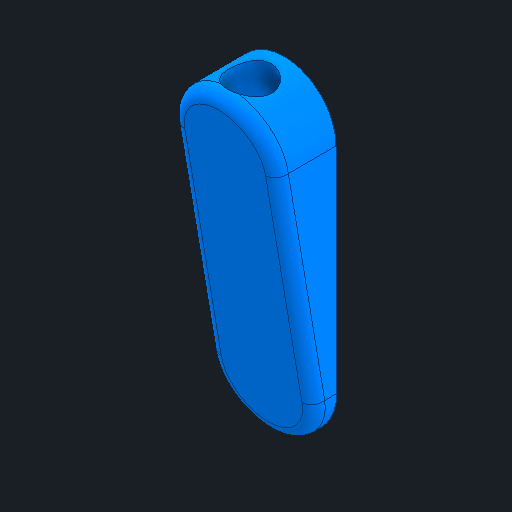
# Autodesk Inventor part: shaft_outlet
Saved by Autodesk Inventor 2023 (Build 270158030, 158C)
## iProperties
Created: 2022-03-28
Part Number: shaft_outlet
Material: Generic
Document SubType Name: Modeling
Designer: kardo
Density: 1 g/cm^3
Appearance: Blue Plastic
Author: kardo
Autodesk Inventor part; units mm, degrees
ref_plane "YZ Plane" through (0, 0, 0) normal (1, 0, 0) x (0, 1, 0)
ref_plane "XZ Plane" through (0, 0, 0) normal (0, 1, 0) x (-1, 0, 0)
ref_plane "XY Plane" through (0, 0, 0) normal (0, 0, 1) x (1, 0, 0)
derived "stencil_frame.ipt"
sketch "sk_drivetrain_profile" plane through (6, 0, 0) normal (1, 0, 0) x (0, 1, 0)
  line L0 (-547.3485, 0) -> (393.091, 0) construction
  line L1 (-363, 4666.1952) -> (-363, -2045.0469) construction
  line L2 (0, 4666.1952) -> (0, -2045.0469) construction
  line L3 (-140.6277, 54.4571) -> (-133.8539, 27.2888)
  line L4 (-395, 0) -> (-331.1194, 3.9071)
  line L5 (-137.2408, 40.8729) -> (-228.5101, 18.117)
  line L6 (-314.0499, 4.9511) -> (-270.6751, 7.604) construction
  line L7 (-270.6751, 7.604) -> (-228.5101, 18.117) construction
  line L8 (-133.8539, 27.2888) -> (-133.8539, 22.2888) construction
  line L9 (-331.1194, 3.9071) -> (-314.0499, 4.9511)
  line L10 (-1246.9714, 4491.7596) -> (383.4376, -2047.4538) construction
  spline S0 degree 2 poles (-314.0499, 4.9511) (-270.6751, 7.604) (-228.5101, 18.117) knots 1 1 1 2 2 2
  line L11 (-229.1821, 20.8126) -> (-137.9129, 43.5685) construction
  line L12 (-136.5687, 38.1773) -> (-227.838, 15.4214) construction
  line L13 (-229.1821, 20.8126) -> (-227.838, 15.4214) construction
  line L14 (0, 21.4767) -> (-254.1001, 20.7404) construction
  line L15 (-55.6943, 22.5153) -> (-309.842, 21.7788) construction
  point P0 (0, 0)
  point P1 (-217.5636, 20.8462)
  point P2 (-205.945, 20.8799)
  point P3 (-201.0754, 22.094)
sketch "sk_prop_shaft_cut" plane through (6, 0, 21.4767) normal (0, -0.0028978, 0.9999958) x (0, -0.9999958, -0.0028978)
  line L0 (229.1831, -4.7781) -> (201.0728, -4.7781)
  line L1 (229.1831, 4.7781) -> (201.0728, 4.7781)
  arc A0 (201.0728, 4.7781) -> (201.0728, -4.7781) centre (201.0728, 0) ccw
  arc A1 (229.1831, -4.7781) -> (229.1831, 4.7781) centre (229.1831, 0) ccw
  point P0 (0.0622, -6)
  point P1 (217.5645, 0)
  point P2 (205.9458, 0)
ref_plane "plane_motor_mount" through (0, -127.05, 0) normal (0, 0.9702957, 0.2419219) x (-1, 0, 0)
derived "parameters_powertrain.ipt"
derived "parameters_frame.ipt"
extrude "lower_plate" add sketch "sk_prop_shaft_cut" along normal blind 1.2
sketch "sk_upper_plate" plane through (6, -229.1856, 22.0126) normal (0, -0.0028978, 0.9999958) x (1, 0, 0)
  line L0 (-4.7781, 28.1103) -> (-4.7781, 0) projected
  arc A0 (-4.7781, 0) -> (4.7781, 0) centre (0, 0) ccw projected
  line L1 (4.7781, 0) -> (4.7781, 28.1103) projected
  arc A1 (4.7781, 28.1103) -> (-4.7781, 28.1103) centre (0, 28.1103) ccw projected
  line L2 (-6.7781, 0) -> (-6.7781, 28.1103)
  arc A2 (6.7781, 28.1103) -> (-6.7781, 28.1103) centre (0, 28.1103) ccw
  line L3 (6.7781, 28.1103) -> (6.7781, 0)
  arc A3 (-6.7781, 0) -> (6.7781, 0) centre (0, 0) ccw
  point P0 (-6, 229.1209)
  dimension "d6" = 2
  constraints: 4 end point, 4 point on circle, 2 centre point, 3 other
  measures "d6" distance between parallel lines of L2 L0
extrude "upper_plate" add sketch "sk_upper_plate" along normal blind 8.89 contours A1 L1 A0 L0 | L2 A2 L3 A3
sketch "sk_trim" plane through (12.7781, -229.1856, 22.0126) normal (1, 0, 0) x (0, 0.0028978, -0.9999958)
  line L0 (-1.9447, -6.7781) -> (-8.89, 34.8885)
  line L1 (0, 0) -> (0, -6.7781) projected
  line L2 (-8.89, 34.8885) -> (-8.89, 28.1103) projected
  line L3 (0, -6.7781) -> (-1.9447, -6.7781)
  line L4 (-1.9447, -6.7781) -> (-8.89, -6.7781)
  line L5 (-8.89, -6.7781) -> (-8.89, 28.1103)
  dimension "d16" = 1.9447
  constraints: 8 end point, 2 collinear, 1 perpendicular
  measures "d16" distance of L1.end L0.start
extrude "trim" cut sketch "sk_trim" against normal through all
sketch "sk_drill" plane through (0, -127.05, 0) normal (0, 0.9702957, 0.2419219) x (-1, 0, 0)
  circle A0 centre (-6, 42.1242) radius 2.7781
  point P0 (0, -30.7362)
  dimension "d9" = 5.5563
  constraints: 1 centre point, 1 coincident
  measures "d9" diameter of A0
extrude "drill" cut sketch "sk_drill" along normal through all both and the other way through all
fillet "Fillet1" radius 1.5 6 edges at (10.7929, -233.9851, 24.2743) (1.2071, -233.9851, 24.2743) (-0.7781, -215.1462, 27.4706) (10.7929, -196.3074, 30.6669) (1.2071, -196.3074, 30.6669) (12.7781, -215.1462, 27.4706)
equation "\"d4\" = shell_thickness"
equation "\"d7\" = 1.6 * prop_shaft_sleeve_od"
equation "\"d16\" = 0.35 * prop_shaft_sleeve_od"
equation "\"d9\" = prop_shaft_sleeve_od"
equation "\"shell_thickness\" = 1.2"
equation "\"prop_shaft_sleeve_od\" = 5.55625"
body "Solid1"
